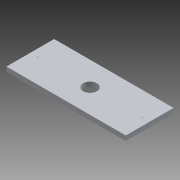
# Autodesk Inventor part: MaterialTest01
Saved by Autodesk Inventor 2013 (Build 170138000, 138)
## iProperties
Created: 2014-07-24
Part Number: MaterialTest01
Material: Generic
Document SubType Name: Modeling
Designer: spichelh
Density: 1 g/cm^3
Author: spichelh
Autodesk Inventor part; units mm, degrees
ref_plane "YZ Plane" through (0, 0, 0) normal (1, 0, 0) x (0, 1, 0)
ref_plane "XZ Plane" through (0, 0, 0) normal (0, 1, 0) x (-1, 0, 0)
ref_plane "XY Plane" through (0, 0, 0) normal (0, 0, 1) x (1, 0, 0)
sketch "Sketch1" plane through (0, 0, 0) normal (0, 0, 1) x (1, 0, 0)
  line L0 (0, 0) -> (25, 0)
  line L1 (25, 0) -> (25, 10)
  line L2 (25, 10) -> (0, 10)
  line L3 (0, 10) -> (0, 0)
  dimension "d0" = 25
  dimension "d1" = 10
  constraints: 8 end point, 2 parallel, 1 horizontal, 1 perpendicular
  measures "d0" distance of L2.end L1.end
  measures "d1" distance of L1.end L0.end
extrude "Extrusion1" add sketch "Sketch1" along normal blind 1
sketch "Sketch2" plane through (0, 0, 1) normal (0, 0, 1) x (1, 0, 0)
  circle A0 centre (12.5, 5) radius 1.45
  line L0 (0, 0) -> (25, 0) projected
  line L1 (0, 10) -> (0, 0) projected
  line L2 (12.5, 0) -> (12.5, 2.5918) construction
  line L3 (25, 0) -> (25, 10) projected
  line L4 (25, 10) -> (0, 10) projected
  line L5 (25, 5) -> (1.9186, 5) construction
  dimension "d4" = 2.9
  constraints: 4 end point, 2 midpoint, 2 parallel, 2 point on line, 1 centre point
  measures "d4" diameter of A0
extrude "Extrusion2" cut sketch "Sketch2" against normal blind 15 contours A0
sketch "Sketch3" plane through (0, 0, 1) normal (0, 0, 1) x (1, 0, 0)
  line L0 (25, 0) -> (25, 10) projected
  line L1 (0, 10) -> (0, 0) projected
  circle A0 centre (23.5, 5) radius 0.1
  circle A1 centre (1.5, 5) radius 0.1
  line L2 (25, 5) -> (0, 5) construction
  dimension "d7" = 0.2
  dimension "d8" = 0.2
  dimension "d9" = 1.5
  dimension "d10" = 1.5
  constraints: 2 centre point, 2 end point, 2 midpoint, 2 point on line
  measures "d7" diameter of A0
  measures "d8" diameter of A1
  measures "d9" distance from line of L1 A1.centre
  measures "d10" distance from line of L0 A0.centre
extrude "Extrusion3" cut sketch "Sketch3" against normal blind 15
body "Solid1"
